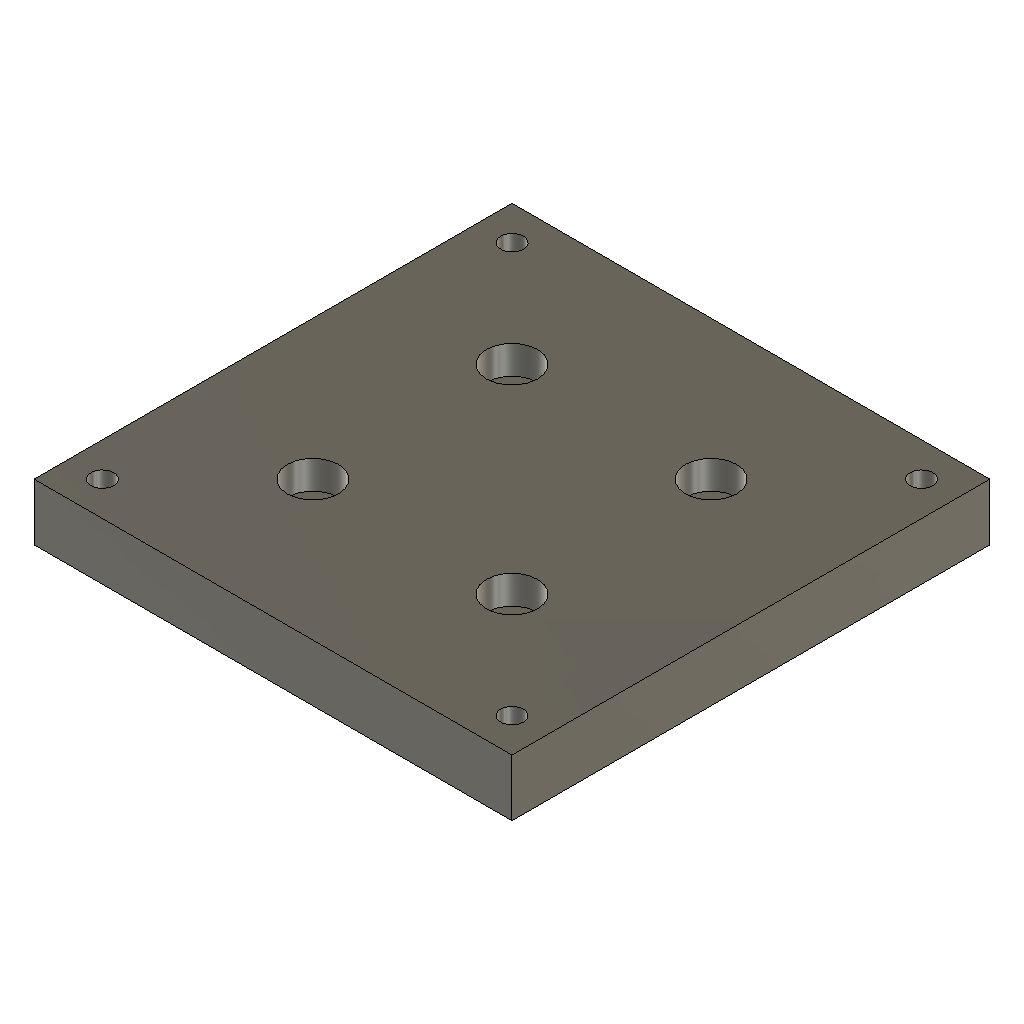
Motor mount (Autodesk Fusion 360 design; units mm, degrees)
Autodesk Fusion 360 part; units mm, degrees
sketch "Base" plane through (0, 0, 0) normal (0, 0, 1) x (1, 0, 0)
  line L0 (0, 0) -> (42, 0)
  line L1 (42, 0) -> (42, 42)
  line L2 (42, 42) -> (0, 42)
  line L3 (0, 42) -> (0, 0)
  dimension "d1" = 42
  dimension "d2" = 42
  constraint horizontal L0
  constraint vertical L1
  constraint horizontal L2
  constraint vertical L3
  constraint coincident L0.start L3.end
  measures "d1" distance of L0.start L0.end
  measures "d2" distance of L0.start L2.end
extrude "Extrude1" add sketch "Base" along normal blind 5
sketch "Mount holes" plane through (0, 0, 5) normal (0, 0, 1) x (-1, 0, 0)
  line L0 (0, -42) -> (0, 0)
  line L1 (0, 0) -> (-42, 0)
  line L2 (-42, 0) -> (-42, -42)
  line L3 (-42, -42) -> (0, -42)
  circle A0 centre (-3, -39) radius 1
  circle A1 centre (-39, -39) radius 1
  circle A2 centre (-3, -3) radius 1
  circle A3 centre (-39, -3) radius 1
  dimension "d8" = 2
  dimension "d9" = 3
  dimension "d10" = 3
  dimension "d11" = 2
  dimension "d12" = 3
  dimension "d13" = 3
  dimension "d14" = 2
  dimension "d15" = 3
  dimension "d16" = 3
  dimension "d17" = 2
  dimension "d18" = 3
  dimension "d19" = 3
  measures "d8" diameter of A0
  measures "d9" distance of L3 A0.centre
  measures "d10" distance of L0 A0.centre
  measures "d11" diameter of A1
  measures "d12" distance of L3 A1.centre
  measures "d13" distance of L2 A1.centre
  measures "d14" diameter of A2
  measures "d15" distance of L0 A2.centre
  measures "d16" distance of L1 A2.centre
  measures "d17" diameter of A3
  measures "d18" distance of L2 A3.centre
  measures "d19" distance of L1 A3.centre
extrude "Extrude2" cut sketch "Mount holes" against normal blind 5 contours A0 | A1 | A2 | A3
sketch "Motor holes" plane through (0, 0, 5) normal (0, 0, 1) x (-1, 0, 0)
  circle A0 centre (-39, -39) radius 1
  circle A1 centre (-3, -3) radius 1
  circle A2 centre (-3, -39) radius 1
  circle A3 centre (-39, -3) radius 1
  line L0 (0, -42) -> (0, 0)
  line L1 (0, 0) -> (-42, 0)
  line L2 (-42, 0) -> (-42, -42)
  line L3 (-42, -42) -> (0, -42)
  circle A4 centre (-12.25, -29.75) radius 1.25
  circle A5 centre (-29.75, -29.75) radius 1.25
  circle A6 centre (-12.25, -12.25) radius 1.25
  circle A7 centre (-29.75, -12.25) radius 1.25
  dimension "d22" = 2.5
  dimension "d23" = 2.5
  dimension "d25" = 12.25
  dimension "d27" = 2.5
  dimension "d28" = 2.5
  dimension "d30" = 12.25
  dimension "d31" = 12.25
  dimension "d32" = 12.25
  dimension "d33" = 12.25
  dimension "d34" = 12.25
  dimension "d35" = 12.25
  dimension "d36" = 12.25
  measures "d22" diameter of A4
  measures "d23" diameter of A5
  measures "d25" distance of L0 A4.centre
  measures "d27" diameter of A6
  measures "d28" diameter of A7
  measures "d30" distance of L0 A6.centre
  measures "d31" distance of L3 A4.centre
  measures "d32" distance of L3 A5.centre
  measures "d33" distance of L1 A6.centre
  measures "d34" distance of L1 A7.centre
  measures "d35" distance of L2 A5.centre
  measures "d36" distance of L2 A7.centre
extrude "Extrude3" cut sketch "Motor holes" against normal blind 5 contours A4 | A5 | A6 | A7
sketch "Fillets" plane through (0, 0, 5) normal (0, 0, 1) x (-1, 0, 0)
  circle A0 centre (-29.75, -29.75) radius 1.25
  circle A1 centre (-12.25, -12.25) radius 1.25
  circle A2 centre (-12.25, -29.75) radius 1.25
  circle A3 centre (-29.75, -12.25) radius 1.25
  circle A4 centre (-39, -39) radius 1
  circle A5 centre (-3, -3) radius 1
  circle A6 centre (-3, -39) radius 1
  circle A7 centre (-39, -3) radius 1
  line L0 (0, -42) -> (0, 0)
  line L1 (0, 0) -> (-42, 0)
  line L2 (-42, 0) -> (-42, -42)
  line L3 (-42, -42) -> (0, -42)
  circle A8 centre (-12.25, -29.75) radius 2.25
  circle A9 centre (-29.75, -29.75) radius 2.25
  circle A10 centre (-12.25, -12.25) radius 2.25
  circle A11 centre (-29.75, -12.25) radius 2.25
  dimension "d39" = 4.5
  dimension "d40" = 4.5
  dimension "d41" = 4.5
  dimension "d42" = 4.5
  constraint concentric A2 A8
  constraint concentric A0 A9
  constraint concentric A1 A10
  constraint concentric A3 A11
  measures "d39" diameter of A8
  measures "d40" diameter of A9
  measures "d41" diameter of A10
  measures "d42" diameter of A11
extrude "Extrude4" cut sketch "Fillets" against normal blind 2.5 contours A8 | A9 | A10 | A11
